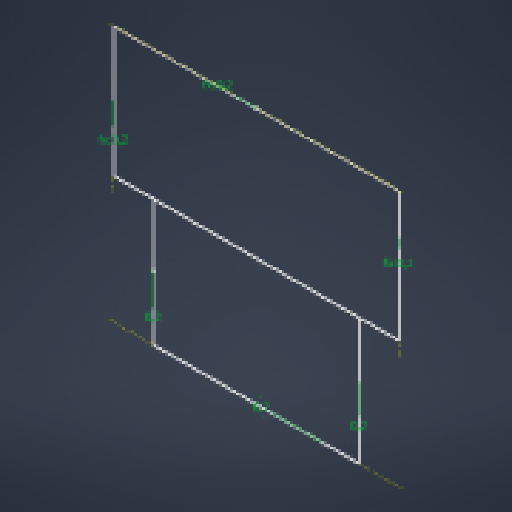
# Autodesk Inventor part: dach
Saved by Autodesk Inventor 2023 (Build 270158000, 158)
## iProperties
Created: 2023-03-22
Part Number: dach
Material: Generic
Document SubType Name: Modeling
Designer: Michał
Density: 1 g/cm^3
Appearance: Default
Author: Michał
Autodesk Inventor part; units mm, degrees
ref_plane "YZ Plane" through (0, 0, 0) normal (1, 0, 0) x (0, 1, 0)
ref_plane "XZ Plane" through (0, 0, 0) normal (0, 1, 0) x (-1, 0, 0)
ref_plane "XY Plane" through (0, 0, 0) normal (0, 0, 1) x (1, 0, 0)
sketch "Sketch1" plane through (0, 0, 0) normal (0, 0, 1) x (1, 0, 0)
  line L0 (24.8, 161.9213) -> (-154.8, 161.9213)
  line L1 (-154.8, 161.9213) -> (-154.8, 70)
  line L2 (-154.8, 70) -> (24.8, 70)
  line L3 (24.8, 70) -> (24.8, 161.9213)
  line L4 (-0.2, 70) -> (-129.8, 70)
  line L5 (-129.8, 70) -> (-129.8, 0.2)
  line L6 (-129.8, 0.2) -> (-0.2, 0.2)
  line L7 (-0.2, 0.2) -> (-0.2, 70)
  line L8 (28, 162.1213) -> (-158, 162.1213) construction
  line L9 (-158, 0) -> (28, 0) construction
  line L10 (-130, 70) -> (-130, 0) construction
  line L11 (0, 70) -> (0, 0) construction
  line L12 (25, 160) -> (25, 70) construction
  line L13 (-155, 160) -> (-155, 70) construction
  line L14 (25, 70) -> (-13, 70) construction
  point P0 (-129.8, 35.1)
  point P1 (-65, 162.1213)
  point P2 (-129.8, 70)
  point P3 (-0.2, 70)
extrude "Extrusion1" add sketch "Sketch1" along normal blind 2
sketch "Sketch2" plane through (0, 0, 2) normal (0, 0, 1) x (1, 0, 0)
  line L0 (16.8, 80) -> (1.598, 80)
  line L1 (1.598, 80) -> (1.598, 88.463)
  line L2 (16.8, 80) -> (16.8, 82.639)
  line L3 (16.8, 82.639) -> (4.231, 82.639)
  line L4 (4.231, 82.639) -> (4.231, 85.831)
  line L5 (4.231, 85.831) -> (16.8, 85.831)
  line L6 (16.8, 85.831) -> (16.8, 91.525)
  line L7 (16.8, 91.525) -> (14.166, 91.525)
  line L8 (14.166, 91.525) -> (14.166, 88.463)
  line L9 (14.166, 88.463) -> (1.598, 88.463)
  line L10 (1.598, 80) -> (-1.709, 80)
  line L11 (-1.709, 80) -> (-1.709, 91.525)
  line L12 (-1.709, 91.525) -> (-4.343, 91.525)
  line L13 (-4.343, 91.525) -> (-4.343, 82.639)
  line L14 (-4.343, 82.639) -> (-15.405, 82.639)
  line L15 (-15.405, 82.639) -> (-15.405, 91.525)
  line L16 (-15.405, 91.525) -> (-18.039, 91.525)
  line L17 (-18.039, 91.525) -> (-18.039, 80)
  line L18 (-18.039, 80) -> (-1.709, 80)
  line L19 (-4.343, 82.639) -> (-8.559, 82.639)
  line L20 (-15.405, 82.639) -> (-11.189, 82.639)
  line L21 (-11.189, 82.639) -> (-11.189, 84.192)
  line L22 (-11.189, 84.192) -> (-8.555, 84.192)
  line L23 (-8.555, 84.192) -> (-8.555, 91.525)
  line L24 (-8.555, 91.525) -> (-11.189, 91.525)
  line L25 (-11.189, 91.525) -> (-11.189, 84.192)
  line L26 (24.8, 70) -> (24.8, 161.9213) projected
  line L27 (-0.2, 70) -> (24.8, 70) projected
  line L28 (-4.2306, 16.2179) -> (-125.7694, 16.1821) construction
  line L29 (-125.7694, 16.1821) -> (-125.778, 45.3709) construction
  line L30 (-125.778, 45.3709) -> (-4.2392, 45.4067) construction
  line L31 (-4.2392, 45.4067) -> (-4.2306, 16.2179) construction
  line L32 (-65, 16.2) -> (-65, 0.2) construction
  line L33 (-129.8, 0.2) -> (-0.2, 0.2) construction
  line L34 (-21.6161, 32.2444) -> (-17.4948, 32.2456)
  line L35 (-17.4948, 32.2456) -> (-17.4939, 28.9044)
  line L36 (-17.4939, 28.9044) -> (-16.2392, 27.6821)
  line L37 (-16.2392, 27.6821) -> (-8.3657, 27.6844)
  line L38 (-8.3657, 27.6844) -> (-8.367, 32.2483)
  line L39 (-8.367, 32.2483) -> (-4.2465, 34.6105)
  line L40 (-4.2465, 34.6105) -> (-4.2418, 18.6105)
  line L41 (-4.2418, 18.6105) -> (-18.5027, 18.6063)
  line L42 (-18.5027, 18.6063) -> (-21.6133, 22.7899)
  line L43 (-21.6133, 22.7899) -> (-19.2532, 25.9632)
  line L44 (-19.2532, 25.9632) -> (-21.6149, 28.334)
  line L45 (-21.6149, 28.334) -> (-21.6161, 32.2444)
  line L46 (-17.3762, 23.0757) -> (-16.2796, 21.6426)
  line L47 (-16.2796, 21.6426) -> (-8.3639, 21.6449)
  line L48 (-8.3639, 21.6449) -> (-8.3648, 24.5856)
  line L49 (-8.3648, 24.5856) -> (-16.2699, 24.5833)
  line L50 (-16.2699, 24.5833) -> (-17.3762, 23.0757)
  line L51 (-41.5361, 29.1397) -> (-38.4382, 32.2394)
  line L52 (-38.4382, 32.2394) -> (-27.0548, 32.2428)
  line L53 (-27.0548, 32.2428) -> (-23.9551, 29.1449)
  line L54 (-23.9551, 29.1449) -> (-23.9529, 21.7035)
  line L55 (-23.9529, 21.7035) -> (-27.0508, 18.6038)
  line L56 (-27.0508, 18.6038) -> (-38.4342, 18.6005)
  line L57 (-38.4342, 18.6005) -> (-41.5339, 21.6984)
  line L58 (-41.5339, 21.6984) -> (-41.5361, 29.1397)
  line L59 (-37.4149, 29.2042) -> (-37.4127, 21.6363)
  line L60 (-37.4127, 21.6363) -> (-28.0741, 21.6391)
  line L61 (-28.0741, 21.6391) -> (-28.0763, 29.2069)
  line L62 (-28.0763, 29.2069) -> (-37.4149, 29.2042)
  line L63 (-61.2881, 28.0588) -> (-58.1905, 32.2547)
  line L64 (-58.1905, 32.2547) -> (-43.7399, 32.259)
  line L65 (-43.7399, 32.259) -> (-43.7359, 18.5989)
  line L66 (-43.7359, 18.5989) -> (-58.1865, 18.5946)
  line L67 (-58.1865, 18.5946) -> (-61.2865, 22.7887)
  line L68 (-61.2865, 22.7887) -> (-59.3479, 25.4243)
  line L69 (-59.3479, 25.4243) -> (-61.2881, 28.0588)
  line L70 (-56.7753, 22.79) -> (-55.7737, 21.652)
  line L71 (-55.7737, 21.652) -> (-47.858, 21.6543)
  line L72 (-47.858, 21.6543) -> (-47.8587, 24.0364)
  line L73 (-47.8587, 24.0364) -> (-55.7744, 24.0341)
  line L74 (-55.7744, 24.0341) -> (-56.7753, 22.79)
  line L75 (-56.7769, 28.0601) -> (-55.7752, 26.8167)
  line L76 (-55.7752, 26.8167) -> (-47.8595, 26.819)
  line L77 (-47.8595, 26.819) -> (-47.8602, 29.2011)
  line L78 (-47.8602, 29.2011) -> (-55.7759, 29.1988)
  line L79 (-55.7759, 29.1988) -> (-56.7769, 28.0601)
  line L80 (-81.0302, 29.1281) -> (-77.9323, 32.2278)
  line L81 (-77.9323, 32.2278) -> (-66.5489, 32.2312)
  line L82 (-66.5489, 32.2312) -> (-63.4491, 29.1333)
  line L83 (-63.4491, 29.1333) -> (-63.4469, 21.6919)
  line L84 (-63.4469, 21.6919) -> (-66.5448, 18.5922)
  line L85 (-66.5448, 18.5922) -> (-77.9282, 18.5888)
  line L86 (-77.9282, 18.5888) -> (-81.028, 21.6867)
  line L87 (-81.028, 21.6867) -> (-81.0302, 29.1281)
  line L88 (-76.909, 29.1925) -> (-76.9067, 21.6247)
  line L89 (-76.9067, 21.6247) -> (-67.5681, 21.6274)
  line L90 (-67.5681, 21.6274) -> (-67.5704, 29.1953)
  line L91 (-67.5704, 29.1953) -> (-76.909, 29.1925)
  line L92 (-87.3552, 32.2461) -> (-83.2347, 34.5873)
  line L93 (-83.2347, 34.5873) -> (-83.2299, 18.5873)
  line L94 (-83.2299, 18.5873) -> (-87.3512, 18.586)
  line L95 (-87.3512, 18.586) -> (-87.3552, 32.2461)
  line L96 (-105.5361, 29.1841) -> (-102.4804, 32.2417)
  line L97 (-102.4804, 32.2417) -> (-89.6951, 32.2454)
  line L98 (-89.6951, 32.2454) -> (-89.6911, 18.5748)
  line L99 (-89.6911, 18.5748) -> (-93.8116, 16.1915)
  line L100 (-93.8116, 16.1915) -> (-93.8154, 29.1876)
  line L101 (-93.8154, 29.1876) -> (-105.5361, 29.1841)
  line L102 (-123.5809, 29.1155) -> (-120.483, 32.2153)
  line L103 (-120.483, 32.2153) -> (-109.0996, 32.2186)
  line L104 (-109.0996, 32.2186) -> (-105.9999, 29.1207)
  line L105 (-105.9999, 29.1207) -> (-105.9977, 21.6794)
  line L106 (-105.9977, 21.6794) -> (-109.0956, 18.5796)
  line L107 (-109.0956, 18.5796) -> (-120.479, 18.5763)
  line L108 (-120.479, 18.5763) -> (-123.5787, 21.6742)
  line L109 (-123.5787, 21.6742) -> (-123.5809, 29.1155)
  line L110 (-119.4597, 29.18) -> (-119.4575, 21.6122)
  line L111 (-119.4575, 21.6122) -> (-110.1189, 21.6149)
  line L112 (-110.1189, 21.6149) -> (-110.1211, 29.1828)
  line L113 (-110.1211, 29.1828) -> (-119.4597, 29.18)
  line L114 (-12.9278, 39.4963) -> (-11.1209, 41.9422)
  line L115 (-11.1209, 41.9422) -> (-6.304, 41.9436)
  line L116 (-6.304, 41.9436) -> (-6.3047, 44.2256)
  line L117 (-6.3047, 44.2256) -> (-4.2444, 45.4067)
  line L118 (-4.2444, 45.4067) -> (-4.2421, 37.4067)
  line L119 (-4.2421, 37.4067) -> (-11.3725, 37.4046)
  line L120 (-11.3725, 37.4046) -> (-12.9278, 39.4963)
  line L121 (-10.804, 39.6393) -> (-10.261, 38.9227)
  line L122 (-10.261, 38.9227) -> (-6.3031, 38.9238)
  line L123 (-6.3031, 38.9238) -> (-6.3036, 40.3942)
  line L124 (-6.3036, 40.3942) -> (-10.2614, 40.393)
  line L125 (-10.2614, 40.393) -> (-10.804, 39.6393)
  line L126 (-21.5243, 42.7033) -> (-19.9964, 44.2321)
  line L127 (-19.9964, 44.2321) -> (-13.6038, 44.2339)
  line L128 (-13.6038, 44.2339) -> (-13.6018, 37.3986)
  line L129 (-13.6018, 37.3986) -> (-15.662, 36.207)
  line L130 (-15.662, 36.207) -> (-15.6639, 42.705)
  line L131 (-15.6639, 42.705) -> (-21.5243, 42.7033)
  line L132 (-30.0359, 44.2291) -> (-27.9648, 44.2297)
  line L133 (-27.9648, 44.2297) -> (-27.9642, 42.264)
  line L134 (-27.9642, 42.264) -> (-23.8166, 42.2652)
  line L135 (-23.8166, 42.2652) -> (-23.8172, 44.2309)
  line L136 (-23.8172, 44.2309) -> (-21.757, 45.4015)
  line L137 (-21.757, 45.4015) -> (-21.755, 38.9298)
  line L138 (-21.755, 38.9298) -> (-23.304, 37.401)
  line L139 (-23.304, 37.401) -> (-28.4845, 37.3995)
  line L140 (-28.4845, 37.3995) -> (-30.0344, 38.9274)
  line L141 (-30.0344, 38.9274) -> (-30.0359, 44.2291)
  line L142 (-27.9638, 40.7567) -> (-27.9632, 38.928)
  line L143 (-27.9632, 38.928) -> (-23.8156, 38.9292)
  line L144 (-23.8156, 38.9292) -> (-23.8162, 40.7579)
  line L145 (-23.8162, 40.7579) -> (-27.9638, 40.7567)
  line L146 (-39.3883, 37.3963) -> (-37.871, 38.9251)
  line L147 (-37.871, 38.9251) -> (-33.286, 38.9264)
  line L148 (-33.286, 38.9264) -> (-33.2871, 42.6998)
  line L149 (-33.2871, 42.6998) -> (-39.1475, 42.6981)
  line L150 (-39.1475, 42.6981) -> (-37.6196, 44.2269)
  line L151 (-37.6196, 44.2269) -> (-32.7764, 44.2283)
  line L152 (-32.7764, 44.2283) -> (-31.2265, 42.7004)
  line L153 (-31.2265, 42.7004) -> (-31.2254, 38.9587)
  line L154 (-31.2254, 38.9587) -> (-32.7744, 37.3983)
  line L155 (-32.7744, 37.3983) -> (-39.3883, 37.3963)
  line L156 (-48.0155, 37.3938) -> (-46.4981, 38.9225)
  line L157 (-46.4981, 38.9225) -> (-41.9131, 38.9239)
  line L158 (-41.9131, 38.9239) -> (-41.9135, 40.1149)
  line L159 (-41.9135, 40.1149) -> (-47.0202, 40.1134)
  line L160 (-47.0202, 40.1134) -> (-45.6293, 41.5051)
  line L161 (-45.6293, 41.5051) -> (-41.9139, 41.5062)
  line L162 (-41.9139, 41.5062) -> (-41.9143, 42.6973)
  line L163 (-41.9143, 42.6973) -> (-47.7746, 42.6956)
  line L164 (-47.7746, 42.6956) -> (-46.2467, 44.2243)
  line L165 (-46.2467, 44.2243) -> (-39.8541, 44.2262)
  line L166 (-39.8541, 44.2262) -> (-39.8521, 37.3962)
  line L167 (-39.8521, 37.3962) -> (-48.0155, 37.3938)
  line L168 (-56.7427, 37.3912) -> (-54.1453, 39.8742)
  line L169 (-54.1453, 39.8742) -> (-56.5281, 42.2556)
  line L170 (-56.5281, 42.2556) -> (-56.5287, 44.2213)
  line L171 (-56.5287, 44.2213) -> (-54.4681, 44.2219)
  line L172 (-54.4681, 44.2219) -> (-54.4676, 42.5566)
  line L173 (-54.4676, 42.5566) -> (-52.9441, 41.0339)
  line L174 (-52.9441, 41.0339) -> (-50.7523, 43.0952)
  line L175 (-50.7523, 43.0952) -> (-50.7527, 44.223)
  line L176 (-50.7527, 44.223) -> (-48.6924, 45.3936)
  line L177 (-48.6924, 45.3936) -> (-48.69, 37.3936)
  line L178 (-48.69, 37.3936) -> (-50.7506, 37.393)
  line L179 (-50.7506, 37.393) -> (-50.7516, 40.7395)
  line L180 (-50.7516, 40.7395) -> (-54.308, 37.3919)
  line L181 (-54.308, 37.3919) -> (-56.7427, 37.3912)
  point P0 (0, 0)
  dimension "d0" = 0.2
  dimension "d1" = 0.2
  dimension "d2" = 0.2
  dimension "d3" = 0.2
  dimension "d4" = 0.2
  dimension "d5" = 0.2
  dimension "d8" = 15.202
  dimension "d9" = 8.463
  dimension "d10" = 2.639
  dimension "d11" = 12.569
  dimension "d12" = 3.192
  dimension "d13" = 5.694
  dimension "d15" = 3.307
  dimension "d17" = 8.886
  dimension "d18" = 11.062
  dimension "d19" = 2.634
  dimension "d20" = 4.216
  dimension "d21" = 4.216
  dimension "d22" = 1.553
  dimension "d23" = 8
  dimension "d24" = 10
  dimension "d25" = 29.1888
  dimension "d26" = 121.5389
  dimension "d27" = 16
  constraints: 54 end point, 15 perpendicular, 7 point on line, 5 collinear, 3 parallel, 2 midpoint, 1 vertical, 2 other
  measures "d8" distance of L0.start L0.end
  measures "d9" distance of L0.end L1.end
  measures "d10" distance of L0.start L2.end
  measures "d11" distance of L2.end L3.end
  measures "d12" distance of L3.end L4.end
  measures "d13" distance of L5.end L6.end
  measures "d15" distance of L0.end L18.end
  measures "d17" distance of L13.start L13.end
  measures "d18" distance of L13.end L15.start
  measures "d19" distance of L15.end L16.end
  measures "d20" distance of L13.end L19.end
  measures "d21" distance of L15.start L21.start
  measures "d22" distance of L21.start L22.start
  measures "d23" distance between parallel lines of L26 L2
  measures "d24" distance between parallel lines of L27 L0
  measures "d25" distance of L30.end L28.start
  measures "d26" distance of L28.start L28.end
  measures "d27" distance of L32.start L32.end
extrude "Extrusion2" cut sketch "Sketch2" against normal blind 1
sketch "Sketch3" plane through (0, 0, 2) normal (0, 0, 1) x (1, 0, 0)
  line L0 (-27.0508, 18.6038) -> (-38.4342, 18.6005) projected
  line L1 (-27.0508, 18.6038) -> (-38.4342, 18.6005)
  line L2 (-41.5339, 21.6984) -> (-41.5361, 29.1397) projected
  line L3 (-38.4342, 18.6005) -> (-41.5339, 21.6984)
  line L4 (-41.5361, 29.1397) -> (-38.4382, 32.2394) projected
  line L5 (-41.5339, 21.6984) -> (-41.5361, 29.1397)
  line L6 (-41.5361, 29.1397) -> (-38.4382, 32.2394)
  line L7 (-38.4382, 32.2394) -> (-27.0548, 32.2428) projected
  line L8 (-38.4382, 32.2394) -> (-27.0548, 32.2428)
  line L9 (-27.0548, 32.2428) -> (-23.9551, 29.1449)
  line L10 (-23.9551, 29.1449) -> (-23.9529, 21.7035) projected
  line L11 (-23.9551, 29.1449) -> (-23.9529, 21.7035)
  line L12 (-23.9529, 21.7035) -> (-27.0508, 18.6038)
  point P0 (0, 0)
  constraints: 16 end point, 4 equal length, 3 perpendicular
extrude "Extrusion3" add sketch "Sketch3" against normal blind 1
sketch "Sketch4" plane through (0, 0, 2) normal (0, 0, 1) x (1, 0, 0)
  circle A0 centre (-32.6757, 25.4216) radius 3.5
  line L0 (-36.6149, 32.24) -> (-28.7404, 32.2423)
  line L1 (-28.7404, 32.2423) -> (-24.8012, 25.424)
  line L2 (-24.8012, 25.424) -> (-28.7364, 18.6033)
  line L3 (-28.7364, 18.6033) -> (-36.6109, 18.601)
  line L4 (-36.6109, 18.601) -> (-40.5501, 25.4193)
  line L5 (-40.5501, 25.4193) -> (-36.6149, 32.24)
  line L6 (-4.2418, 18.6105) -> (-18.5027, 18.6063) projected
  line L7 (-21.6161, 32.2444) -> (-17.4948, 32.2456) projected
  line L8 (-40.5501, 25.4193) -> (-43.7379, 25.4289) construction
  line L9 (-43.7399, 32.259) -> (-43.7359, 18.5989) construction
  line L10 (-24.8012, 25.424) -> (-21.614, 25.3623) construction
  line L11 (-21.6149, 28.334) -> (-21.6161, 32.2444) construction
  line L12 (-43.7399, 32.259) -> (-43.7359, 18.5989) construction
  point P0 (0, 0)
  dimension "d32" = 7
  constraints: 16 end point, 3 midpoint, 2 collinear, 2 point on line, 1 centre point, 1 coincident, 1 equal length, 13 other
  measures "d32" diameter of A0
extrude "Extrusion4" cut sketch "Sketch4" against normal blind 1
sketch "Sketch5" plane through (0, 0, 2) normal (0, 0, 1) x (1, 0, 0)
  line L0 (-123, 146) -> (-116, 146) projected
  line L1 (-123, 157) -> (-116, 157) projected
  line L2 (-14, 157) -> (-7, 157) projected
  line L3 (-7, 146) -> (-14, 146) projected
  line L4 (-138, 157) -> (-138, 145) projected
  line L5 (-138, 157) -> (-134.042, 157) projected
  line L6 (-131.958, 157) -> (-134.042, 157) projected
  line L7 (-131.958, 157) -> (-129, 157) projected
  line L8 (-129, 145) -> (-129, 157) projected
  line L9 (-138, 145) -> (-129, 145) projected
  line L10 (-7, 157) -> (-7, 146)
  line L11 (-14, 146) -> (-14, 157)
  line L12 (-116, 157) -> (-116, 146)
  line L13 (-123, 146) -> (-123, 157)
  line L14 (-116, 143) -> (-126.5, 143) projected
  line L15 (-124.5636, 128) -> (-116, 128) projected
  line L16 (-116, 128) -> (-126.5, 128) projected
  line L17 (-126.5, 128) -> (-126.5, 143)
  line L18 (-116, 143) -> (-116, 128)
  point P0 (0, 0)
  constraints: 12 end point, 3 parallel, 3 vertical
extrude "Extrusion5" cut sketch "Sketch5" against normal through all
equation "\"d3\" = d0"
equation "\"d4\" = d0"
equation "\"d5\" = d0"
body "Solid1"
